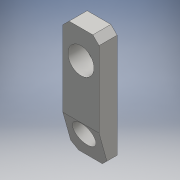
# Autodesk Inventor part: HeadbarClamp
Saved by Autodesk Inventor 2016 (Build 200138000, 138)
## iProperties
Created: 2015-11-18
Part Number: HeadbarClamp
Material: Generic
Document SubType Name: Modeling
Designer: Vervaeke-Lab
Density: 1 g/cm^3
Appearance: Default
Author: Vervaeke-Lab
Autodesk Inventor part; units mm, degrees
ref_plane "YZ Plane" through (0, 0, 0) normal (1, 0, 0) x (0, 1, 0)
ref_plane "XZ Plane" through (0, 0, 0) normal (0, 1, 0) x (-1, 0, 0)
sketch "Sketch1" plane through (0, 0, 0) normal (0, 1, 0) x (-1, 0, 0)
  line L0 (0, 0) -> (6.4, 0)
  line L1 (6.4, 0) -> (6.4, -20.6)
  line L2 (6.4, -20.6) -> (0, -20.6)
  line L3 (0, -20.6) -> (0, 0)
  point P0 (3.2, -7.9)
  dimension "d0" = 6.4
  dimension "d1" = 20.6
  constraints: 8 end point, 2 parallel, 1 horizontal, 1 perpendicular
  measures "d0" distance of L1.end L2.end
  measures "d1" distance of L0.end L1.end
extrude "Extrusion1" add sketch "Sketch1" along normal blind 3.2
sketch "Sketch3" plane through (0, 0, 0) normal (0, -1, 0) x (1, 0, 0)
  point P0 (0, 0)
  point P1 (-3.2, -5)
hole "Hole1" at (-3.2, 0, -5) direction (0, 1, 0) diameter 4.6 end through all
chamfer "Chamfer1" distance 1.1 angle 45 1 edges at (0, 1.6, 0)
chamfer "Chamfer2" distance 1.1 angle 45 1 edges at (-6.4, 1.6, 0)
chamfer "Chamfer3" distance 1.1 angle 45 1 edges at (-6.4, 1.6, -20.6)
chamfer "Chamfer4" distance 1.1 angle 45 1 edges at (0, 1.6, -20.6)
sketch "Sketch5" plane through (0, 0, 0) normal (1, 0, 0) x (0, 1, 0)
  line L0 (3.2, -20.6) -> (0, -20.6) projected
  line L1 (0, -20.6) -> (0, -14.5)
  line L2 (0, -1.1) -> (0, -19.5) projected
  line L3 (0, -20.6) -> (1.7, -20.6)
  line L4 (1.7, -20.6) -> (0, -14.5)
  point P0 (0, 0)
  dimension "d26" = 6.1
  dimension "d27" = 1.7
  constraints: 6 end point, 2 point on line
  measures "d26" distance of L0.end L1.end
  measures "d27" distance of L0.end L3.end
extrude "Extrusion3" cut sketch "Sketch5" against normal through all
ref_plane "Work Plane1" through (-6.4, 0, -14.5) normal (0, -0.9633, -0.2685) x (1, 0, 0)
sketch "Sketch11" plane through (-6.4, 0, -14.5) normal (0, -0.9633, -0.2685) x (1, 0, 0)
  circle A0 centre (3.2, -2.1) radius 2.01
  line L0 (0, 0) -> (6.4, 0) projected
  point P0 (6.4, 13.9677)
  dimension "d31" = 4.02
  dimension "d34" = 2.1
  constraints: 1 centre point
  measures "d31" diameter of A0
  measures "d34" distance from line of A0.centre L0
extrude "Extrusion4" cut sketch "Sketch11" along normal mid plane 4.2
body "Solid1"
